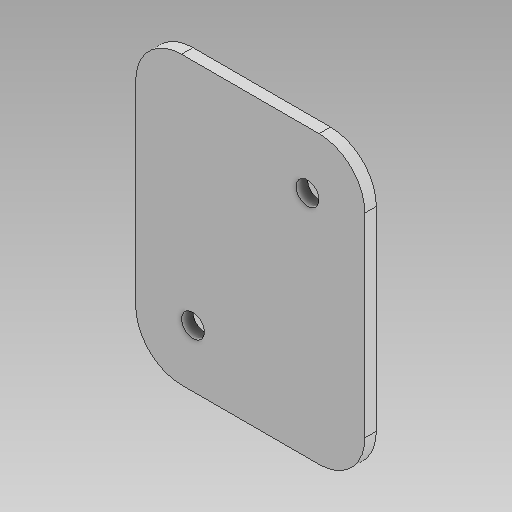
# Autodesk Inventor part: base
Saved by Autodesk Inventor 2025 (Build 290162000, 162)
## iProperties
Created: 2024-09-22
Part Number: base
Material: 일반
Document SubType Name: Modeling
Designer: OSB
Density: 1 g/cm^3
Appearance: 기본값
Author: OSB
Autodesk Inventor part; units mm, degrees
ref_plane "YZ Plane" through (0, 0, 0) normal (1, 0, 0) x (0, 1, 0)
ref_plane "XZ Plane" through (0, 0, 0) normal (0, 1, 0) x (-1, 0, 0)
ref_plane "XY Plane" through (0, 0, 0) normal (0, 0, 1) x (1, 0, 0)
sketch "스케치1" plane through (0, 0, 0) normal (0, 0, 1) x (1, 0, 0)
  circle A0 centre (0, 0) radius 5
  circle A1 centre (50, 75) radius 5
  line L0 (-5, -25) -> (55, -25)
  line L1 (75, -5) -> (75, 80)
  line L2 (55, 100) -> (-5, 100)
  line L3 (-25, 80) -> (-25, -5)
  arc A2 (55, -25) -> (75, -5) centre (55, -5) ccw
  arc A3 (-25, -5) -> (-5, -25) centre (-5, -5) ccw
  arc A4 (-5, 100) -> (-25, 80) centre (-5, 80) ccw
  arc A5 (75, 80) -> (55, 100) centre (55, 80) ccw
  point P0 (-25, -25)
  point P1 (75, 100)
  point P2 (75, -25)
  point P3 (-25, 100)
  dimension "d0" = 10
  dimension "d1" = 10
  dimension "d2" = 50
  dimension "d3" = 75
  dimension "d4" = 25
  dimension "d5" = 25
  dimension "d6" = 25
  dimension "d7" = 25
  dimension "d10" = 20
  constraints: 8 end point, 8 point on circle, 8 point on line, 8 tangent, 6 centre point, 3 equal radius, 2 parallel, 1 coincident, 1 horizontal, 1 perpendicular
  measures "d0" diameter of A0
  measures "d1" diameter of A1
  measures "d2" horizontal distance of point (0, 0) A1.centre
  measures "d3" vertical distance of point (0, 0) A1.centre
  measures "d4" distance from line of L3 point (0, 0)
  measures "d5" distance from line of L0 point (0, 0)
  measures "d6" distance from line of L1 A1.centre
  measures "d7" distance from line of L2 A1.centre
  measures "d10" radius of A2
extrude "돌출1" add sketch "스케치1" along normal blind 5
